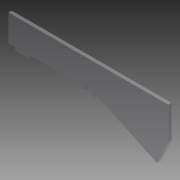
# Autodesk Inventor part: Side Wall
Saved by Autodesk Inventor 2013 (Build 170138000, 138)
## iProperties
Created: 2013-01-28
Part Number: Side Wall
Material: Polycarbonate, Clear
Document SubType Name: Modeling
Designer: Andrew Toennies
Density: 1.2 g/cm^3
Mass: 19.2453 g
Surface Area: 113.791 cm^2
Volume: 16.0378 cm^3
Author: Andrew Toennies
Autodesk Inventor part; units mm, degrees
ref_plane "YZ Plane" through (0, 0, 0) normal (1, 0, 0) x (0, 1, 0)
ref_plane "XZ Plane" through (0, 0, 0) normal (0, 1, 0) x (-1, 0, 0)
ref_plane "XY Plane" through (0, 0, 0) normal (0, 0, 1) x (1, 0, 0)
sketch "Sketch1" plane through (0, 0, 0) normal (0, 0, 1) x (1, 0, 0)
  line L0 (0, 0) -> (0, 25.4)
  line L1 (0, 25.4) -> (79.375, 25.4)
  line L2 (79.375, 25.4) -> (79.375, 0)
  line L3 (79.375, 0) -> (73.025, 0)
  line L4 (73.025, 0) -> (73.025, -3.175)
  line L5 (73.025, -3.175) -> (60.325, -3.175)
  line L6 (60.325, -3.175) -> (60.325, 0)
  line L7 (0, 0) -> (6.35, 0)
  line L8 (6.35, 0) -> (6.35, -3.175)
  line L9 (6.35, -3.175) -> (19.05, -3.175)
  line L10 (19.05, -3.175) -> (19.05, 0)
  line L11 (19.05, 0) -> (60.325, 0)
  dimension "d0" = 25.4
  dimension "d1" = 79.375
  dimension "d2" = 6.35
  dimension "d4" = 3.175
  dimension "d5" = 12.7
  dimension "d6" = 6.35
  dimension "d7" = 3.175
  dimension "d8" = 12.7
  dimension "d9" = 25.4
  dimension "d10" = 25.4
  constraints: 24 end point, 8 perpendicular, 3 parallel, 1 vertical
  measures "d0" distance of L0.start L0.end
  measures "d1" distance of L0.end L1.end
  measures "d2" distance of L2.end L3.end
  measures "d4" distance of L3.end L4.end
  measures "d5" distance of L4.end L5.end
  measures "d6" distance of L0.start L7.end
  measures "d7" distance of L7.end L8.end
  measures "d8" distance of L8.end L9.end
  measures "d9" distance between parallel lines of L1 L11
  measures "d10" distance between parallel lines of L1 L3
extrude "Extrusion1" add sketch "Sketch1" along normal blind 3.175
sketch "Sketch2" plane through (0, 0, 3.175) normal (0, 0, 1) x (1, 0, 0)
  line L0 (141.5184, -31.3531) -> (142.8602, -28.4755) projected
  line L1 (125.5951, -20.4247) -> (137.1052, -25.7919) projected
  line L2 (124.2533, -23.3022) -> (125.5951, -20.4247) projected
  line L3 (135.7634, -28.6694) -> (124.2533, -23.3022) projected
  line L4 (137.1052, -25.7919) -> (135.7634, -28.6694) projected
  line L5 (101.233, -12.5677) -> (89.7229, -7.2004) projected
  line L6 (102.5748, -9.6902) -> (101.233, -12.5677) projected
  line L7 (91.0647, -4.3229) -> (102.5748, -9.6902) projected
  line L8 (89.7229, -7.2004) -> (91.0647, -4.3229) projected
  line L9 (83.9679, -4.5168) -> (85.3097, -1.6393) projected
  line L10 (79.375, 0) -> (79.375, -3.175) projected
  line L11 (79.375, -3.175) -> (81.0903, -3.175)
  line L12 (83.9679, -4.5168) -> (81.0903, -3.175)
  line L13 (79.375, -3.175) -> (79.375, 25.4)
  line L14 (79.375, 25.4) -> (87.4253, 25.4)
  line L15 (83.9679, -4.5168) -> (85.3097, -1.6393)
  line L16 (85.3097, -1.6393) -> (91.0647, -4.3229)
  line L17 (91.0647, -4.3229) -> (89.7229, -7.2004)
  line L18 (89.7229, -7.2004) -> (101.233, -12.5677)
  line L19 (102.5748, -9.6902) -> (101.233, -12.5677)
  line L20 (102.5748, -9.6902) -> (125.5951, -20.4247)
  line L21 (125.5951, -20.4247) -> (124.2533, -23.3022)
  line L22 (124.2533, -23.3022) -> (135.7634, -28.6694)
  line L23 (137.1052, -25.7919) -> (135.7634, -28.6694)
  line L24 (142.8602, -28.4755) -> (137.0616, -25.7716)
  line L25 (142.8602, -28.4755) -> (153.5947, -5.4553)
  line L26 (79.375, 25.4) -> (0, 25.4) projected
  line L27 (87.4253, 25.4) -> (153.5947, 25.4)
  line L28 (153.5947, 25.4) -> (153.5947, -5.4553)
  dimension "d13" = 25.4
  constraints: 34 end point, 11 perpendicular, 5 collinear, 1 point on line
  measures "d13" distance of L0.end L25.end
extrude "Extrusion2" add sketch "Sketch2" against normal blind 3.175 contours L20 L7 L16 L9 L12 L11 L10 L13 L14 L27 L28 L25 L24 L1
body "Solid1"
